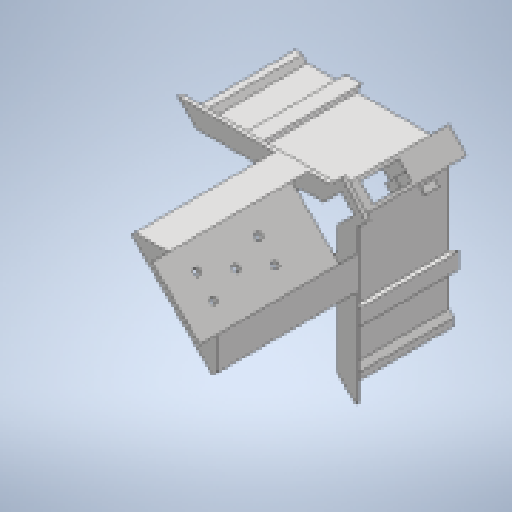
# Autodesk Inventor part: Kicker
Saved by Autodesk Inventor 2025.1 (Build 291241000, 241)
## iProperties
Created: 2025-05-21
Part Number: Kicker
Material: Generic
Document SubType Name: Modeling
Designer: User
Density: 1 g/cm^3
Appearance: Default
Author: User
Autodesk Inventor part; units mm, degrees
ref_plane "YZ Plane" through (0, 0, 0) normal (1, 0, 0) x (0, 1, 0)
sketch "Sketch1" plane through (0, 0, 0) normal (0, 0, 1) x (1, 0, 0)
  line L0 (-95.1092, -28.5) -> (-84.7092, -28.5) projected
  line L1 (-92.4092, -34) -> (-95.1092, -28.5) projected
  line L2 (-84.7092, -28.5) -> (-87.4092, -34) projected
  line L3 (-44.9455, -34) -> (-87.4092, -34) projected
  line L4 (-44.9455, -34) -> (-34.1024, -23.1569) projected
  line L5 (-34.1024, -23.1569) -> (-23.5803, -34.5602) projected
  line L6 (-34, -44.9799) -> (-23.5803, -34.5602) projected
  line L7 (-34, -87.4092) -> (-34, -44.9799) projected
  line L8 (-34, -87.4092) -> (-28.5, -84.7092) projected
  line L9 (-28.5, -84.7092) -> (-28.5, -95.1092) projected
  line L10 (-28.5, -95.1092) -> (-34, -92.4092) projected
  line L11 (-131.4592, -24.1043) -> (-125.0635, -30.5) projected
  line L12 (-121.2635, -34.3) -> (-91.9277, -34.3)
  line L13 (-91.9277, -34.3) -> (-94.6277, -28.8)
  line L14 (-94.6277, -28.8) -> (-85.1907, -28.8)
  line L15 (-85.1907, -28.8) -> (-87.8907, -34.3)
  line L16 (-87.8907, -34.3) -> (-44.8212, -34.3)
  line L17 (-44.8212, -34.3) -> (-34.111, -23.5898)
  line L18 (-34.111, -23.5898) -> (-23.9962, -34.5518)
  line L19 (-23.9962, -34.5518) -> (-34.3, -44.8556)
  line L20 (-34.3, -44.8556) -> (-34.3, -87.8907)
  line L21 (-34.3, -87.8907) -> (-28.8, -85.1907)
  line L22 (-28.8, -85.1907) -> (-28.8, -94.6277)
  line L23 (-28.8, -94.6277) -> (-34.3, -91.9277)
  line L24 (-34.3, -91.9277) -> (-34.3, -121.2635)
  line L25 (-36.8, -118.7635) -> (-36.8, -87.9155)
  line L26 (-36.8, -91.9029) -> (-36.8, -44.5272)
  line L27 (-44.4928, -36.8) -> (-91.9029, -36.8)
  line L28 (-87.9155, -36.8) -> (-118.7635, -36.8)
  line L29 (-34.3, -121.2635) -> (-36.8, -118.7635)
  line L30 (-121.2635, -34.3) -> (-118.7635, -36.8)
  line L31 (-43.9928, -36.3) -> (-34.169, -26.4762)
  line L32 (-34.169, -26.4762) -> (-26.769, -34.4961)
  line L33 (-26.769, -34.4961) -> (-36.3, -44.0272)
  line L34 (-43.9928, -36.3) -> (-44.4928, -36.8)
  line L35 (-36.3, -44.0272) -> (-36.8, -44.5272)
  point P0 (0, 0)
  dimension "d1" = 2.5
  constraints: 48 end point, 3 point on line, 1 parallel, 10 other
  measures "d1" distance between parallel lines of L12 L28
ref_plane "Work Plane1" through (-125.0635, -34, -60.4376) normal (0, 0, -1) x (0, 1, 0)
extrude "Extrusion1" add sketch "Sketch1" against normal up to surface (60.4376 mm away)
sketch "Sketch2" plane through (0, 0, 0) normal (0, 0, 1) x (1, 0, 0)
  line L0 (-91.9277, -34.3) -> (-121.2635, -34.3) projected
  line L1 (-94.6277, -28.8) -> (-91.9277, -34.3) projected
  line L2 (-85.1907, -28.8) -> (-94.6277, -28.8) projected
  line L3 (-87.8907, -34.3) -> (-85.1907, -28.8) projected
  line L4 (-44.8212, -34.3) -> (-87.8907, -34.3) projected
  line L5 (-34.111, -23.5898) -> (-44.8212, -34.3) projected
  line L6 (-23.9962, -34.5518) -> (-34.111, -23.5898) projected
  line L7 (-34.3, -44.8556) -> (-23.9962, -34.5518) projected
  line L8 (-34.3, -87.8907) -> (-34.3, -44.8556) projected
  line L9 (-28.8, -85.1907) -> (-34.3, -87.8907) projected
  line L10 (-28.8, -94.6277) -> (-28.8, -85.1907) projected
  line L11 (-34.3, -91.9277) -> (-28.8, -94.6277) projected
  line L12 (-34.3, -121.2635) -> (-34.3, -91.9277) projected
  line L13 (-31.3, -121.2635) -> (-31.3, -96.7425)
  line L14 (-31.3, -96.7425) -> (-25.8, -99.4425)
  line L15 (-25.8, -99.4425) -> (-25.8, -80.376)
  line L16 (-25.8, -80.376) -> (-31.3, -83.076)
  line L17 (-31.3, -83.076) -> (-31.3, -46.0983)
  line L18 (-31.3, -46.0983) -> (-19.8371, -34.6354)
  line L19 (-19.8371, -34.6354) -> (-34.0241, -19.2602)
  line L20 (-34.0241, -19.2602) -> (-46.0639, -31.3)
  line L21 (-46.0639, -31.3) -> (-83.076, -31.3)
  line L22 (-83.076, -31.3) -> (-80.376, -25.8)
  line L23 (-80.376, -25.8) -> (-99.4425, -25.8)
  line L24 (-99.4425, -25.8) -> (-96.7425, -31.3)
  line L25 (-96.7425, -31.3) -> (-121.2635, -31.3)
  line L26 (-131.4592, -24.1043) -> (-125.0635, -30.5) projected
  line L27 (-121.2635, -31.3) -> (-124.2635, -31.3)
  line L28 (-124.2635, -31.3) -> (-118.7635, -36.8)
  line L29 (-118.7635, -36.8) -> (-44.4928, -36.8) projected
  line L30 (-118.7635, -36.8) -> (-44.4928, -36.8)
  line L31 (-34.169, -26.4762) -> (-26.769, -34.4961) projected
  line L32 (-44.4928, -36.8) -> (-34.169, -26.4762)
  line L33 (-34.169, -26.4762) -> (-26.769, -34.4961)
  line L34 (-26.769, -34.4961) -> (-36.7828, -44.51)
  line L35 (-36.7828, -44.51) -> (-36.7828, -118.7807)
  line L36 (-36.7828, -118.7807) -> (-31.3, -124.2635)
  line L37 (-31.3, -124.2635) -> (-31.3, -121.2635)
  point P0 (0, 0)
  point P1 (-121.5635, -34)
  dimension "d5" = 3
  constraints: 45 end point, 3 point on line, 2 horizontal, 2 parallel, 2 perpendicular, 1 collinear, 12 other
  measures "d5" distance between parallel lines of L12 L13
extrude "Extrusion2" add sketch "Sketch2" along normal blind 2.5
sketch "Sketch3" plane through (0, 0, 0) normal (0, 0, -1) x (-1, 0, 0)
  line L0 (124.2635, -31.3) -> (121.2635, -34.3) projected
  line L1 (96.7425, -31.3) -> (124.2635, -31.3) projected
  line L2 (91.9277, -34.3) -> (121.2635, -34.3) projected
  line L3 (116.6137, -34) -> (120.1137, -30.5) projected
  line L4 (117.0209, -34.3) -> (120.0209, -31.3)
  line L5 (30.5, -120.1137) -> (34, -116.6137) projected
  line L6 (31.3, -120.0209) -> (34.3, -117.0209)
  line L7 (34.3, -121.2635) -> (34.3, -91.9277) projected
  line L8 (34.3, -121.2635) -> (31.3, -124.2635) projected
  line L9 (31.3, -124.2635) -> (31.3, -96.7425) projected
  point P0 (0, 0)
  dimension "d8" = 0.5
  dimension "d9" = 0.5
  constraints: 4 end point, 4 point on line, 2 parallel
  measures "d8" distance between parallel lines of L3 L4
  measures "d9" distance between parallel lines of L5 L6
extrude "Extrusion3" add sketch "Sketch3" along normal up to surface (60.4376 mm away)
fillet "Fillet1" radius 4 4 edges at (-118.7635, -36.8, -30.2188) (-118.7635, -36.8, 1.25) (-36.8, -118.7635, -30.2188) (-36.7828, -118.7807, 1.25)
sketch "Sketch4" plane through (0, 0, 2.5) normal (0, 0, 1) x (1, 0, 0)
  line L0 (-46.0639, -31.3) -> (-83.076, -31.3) projected
  line L1 (-96.7425, -31.3) -> (-124.2635, -31.3) projected
  line L2 (-80.376, -25.8) -> (-99.4425, -25.8) projected
  line L3 (-83.076, -31.3) -> (-80.376, -25.8) projected
  line L4 (-99.4425, -25.8) -> (-96.7425, -31.3) projected
  line L5 (-34.0241, -19.2602) -> (-46.0639, -31.3) projected
  line L6 (-124.2635, -31.3) -> (-119.9351, -35.6284) projected
  line L7 (-131.4592, -24.1043) -> (-125.0635, -30.5) projected
  line L8 (-99.4425, -25.8) -> (-129.7635, -25.8)
  line L9 (-129.7635, -25.8) -> (-124.2635, -31.3)
  line L10 (-124.2635, -31.3) -> (-96.7425, -31.3)
  line L11 (-91.9277, -34.3) -> (-117.0209, -34.3) projected
  line L12 (-96.7425, -31.3) -> (-99.4425, -25.8)
  line L13 (-83.076, -31.3) -> (-80.376, -25.8)
  line L14 (-80.376, -25.8) -> (-99.4425, -25.8) projected
  line L15 (-80.376, -25.8) -> (-40.5639, -25.8)
  line L16 (-40.5639, -25.8) -> (-46.0639, -31.3)
  line L17 (-46.0639, -31.3) -> (-83.076, -31.3) projected
  line L18 (-46.0639, -31.3) -> (-83.076, -31.3)
  line L19 (-83.076, -31.3) -> (-80.376, -25.8) projected
  line L20 (-83.076, -31.3) -> (-80.376, -25.8)
  line L21 (-25.8, -80.376) -> (-31.3, -83.076) projected
  line L22 (-31.3, -83.076) -> (-31.3, -46.0983) projected
  line L23 (-31.3, -46.0983) -> (-19.8371, -34.6354) projected
  line L24 (-31.3, -96.7425) -> (-25.8, -99.4425) projected
  line L25 (-31.3, -124.2635) -> (-31.3, -96.7425) projected
  line L26 (-35.6112, -119.9523) -> (-31.3, -124.2635) projected
  line L27 (-30.5, -125.0635) -> (-24.1043, -131.4592) projected
  line L28 (-25.8, -99.4425) -> (-25.8, -129.7635)
  line L29 (-25.8, -129.7635) -> (-31.3, -124.2635)
  line L30 (-31.3, -124.2635) -> (-31.3, -96.7425)
  line L31 (-31.3, -96.7425) -> (-25.8, -99.4425)
  line L32 (-25.8, -80.376) -> (-31.3, -83.076)
  line L33 (-31.3, -83.076) -> (-31.3, -46.0983)
  line L34 (-25.8, -80.376) -> (-25.8, -40.5983)
  line L35 (-25.8, -40.5983) -> (-31.3, -46.0983)
  line L36 (-34.3, -44.8556) -> (-23.9962, -34.5518) projected
  line L37 (-31.3, -46.0983) -> (-31.3, -83.076)
  line L38 (-34.3, -87.8907) -> (-34.3, -44.8556) projected
  line L39 (-25.8, -80.376) -> (-31.3, -83.076)
  point P0 (0, 0)
  constraints: 38 end point, 7 collinear, 5 parallel, 5 point on line, 2 vertical, 1 horizontal
extrude "Extrusion4" add sketch "Sketch4" against normal up to surface (2.5 mm away)
sketch "Sketch5" plane through (0, 0, 2.5) normal (0, 0, 1) x (1, 0, 0)
  line L0 (-56.2709, -42.724) -> (-60.815, -38.18) projected
  line L1 (-56.235, -42.7599) -> (-42.5671, -56.4279) projected
  line L2 (-37.9871, -61.0078) -> (-42.5312, -56.4638) projected
  line L3 (-37.9871, -61.0078) -> (-60.815, -38.18)
  line L4 (-60.815, -38.18) -> (-62.9363, -40.3013)
  line L5 (-62.9363, -40.3013) -> (-40.1085, -63.1291)
  line L6 (-40.1085, -63.1291) -> (-37.9871, -61.0078)
  point P0 (0, 0)
  dimension "d15" = 3
  constraints: 8 end point, 2 parallel, 1 collinear, 1 perpendicular
  measures "d15" distance of L4.end L0.end
ref_plane "Work Plane2" through (-59.6026, -59.7955, 84.008) normal (0, 0, 1) x (0.7071068, -0.7071068, 0)
extrude "Extrusion5" add sketch "Sketch5" along normal up to surface (81.508 mm away)
sketch "Sketch6" plane through (-62.9363, -40.3013, 84.008) normal (-0.7071068, -0.7071068, 0) x (-0.7071068, 0.7071068, 0)
  spline S0 degree 3 poles (-18.1417, 35.1354) (-18.1417, 35.3868) (-18.0914, 35.6547) (-17.8872, 36.1474) (-17.7334, 36.3722) (-17.3785, 36.7271) (-17.1537, 36.8809) (-16.661, 37.0851) (-16.3931, 37.1354) (-15.8903, 37.1354) (-15.6224, 37.0851) (-15.1297, 36.8809) (-14.9049, 36.7271) (-14.55, 36.3722) (-14.3962, 36.1474) (-14.192, 35.6547) (-14.1417, 35.3868) (-14.1417, 34.884) (-14.192, 34.6161) (-14.3962, 34.1234) (-14.55, 33.8986) (-14.9049, 33.5437) (-15.1297, 33.3899) (-15.6224, 33.1857) (-15.8903, 33.1354) (-16.3931, 33.1354) (-16.661, 33.1857) (-17.1537, 33.3899) (-17.3785, 33.5437) (-17.7334, 33.8986) (-17.8872, 34.1234) (-18.0914, 34.6161) (-18.1417, 34.884) (-18.1417, 35.1354) knots 0 0 0 0 0.07541 0.07541 0.150821 0.150821 0.226231 0.226231 0.30164 0.30164 0.37705 0.37705 0.45246 0.45246 0.52787 0.52787 0.603281 0.603281 0.678691 0.678691 0.754101 0.754101 0.829511 0.829511 0.904921 0.904921 0.980331 0.980331 1.055741 1.055741 1.131151 1.131151 1.206562 1.206562 1.206562 1.206562 projected
  circle A0 centre (-9.2456, 17.1903) radius 2 projected
  circle A1 centre (-23.0378, 17.1903) radius 2 projected
  circle A2 centre (-23.0378, 53.0805) radius 2 projected
  circle A3 centre (-9.2456, 53.0805) radius 2 projected
  point P0 (-16.0053, 84.008)
  point P1 (-18.1417, 35.1354)
extrude "Extrusion6" cut sketch "Sketch6" against normal blind 10
sketch "Sketch7" plane through (-37.9871, -61.0078, 84.008) normal (0, 0, 1) x (0.7071068, 0.7071068, 0)
  line L0 (-40, -57.2352) -> (23.0493, 5.8141) projected
  line L1 (23.0737, 26.7177) -> (-40, 89.7914) projected
  line L2 (0, 32.2834) -> (0, 0) projected
  line L3 (-3, 0) -> (-3, 32.2834) projected
  line L4 (0, 49.7914) -> (0, -17.2352)
  line L5 (0, -17.2352) -> (-3, -17.2352)
  line L6 (-3, -17.2352) -> (-3, 49.7914)
  line L7 (-3, 49.7914) -> (0, 49.7914)
  line L8 (-3, 32.2834) -> (0, 32.2834) projected
  line L9 (0, 32.2834) -> (-3, 32.2834)
  line L10 (-3, 32.2834) -> (-3, 0)
  line L11 (0, 0) -> (-3, 0) projected
  line L12 (0, 0) -> (-3, 0)
  point P0 (70, 16.2781)
  point P1 (0, 0)
  point P2 (-3, 0)
  point P3 (-3, 32.2834)
  point P4 (0, 32.2834)
  constraints: 14 end point, 3 equal length, 3 perpendicular, 2 point on line, 1 vertical
extrude "Extrusion7" add sketch "Sketch7" against normal up to surface (81.508 mm away) contours L8 L6 L7 L4 | L4 L5 L6 L11
sketch "Sketch8" plane through (-25.8, -73.1949, 84.008) normal (0, 0, 1) x (0.7071068, 0.7071068, 0)
  arc A0 (7.1422, 21.3881) -> (31.9738, 21.3881) centre (19.558, 33.3769) ccw projected
  arc A1 (29.0311, 47.8041) -> (10.0849, 47.8041) centre (19.558, 33.3769) ccw projected
  line L0 (0, 0) -> (0, 67.0266) projected
  line L1 (19.558, 16.1176) -> (0, 16.1176)
  line L2 (19.558, 50.6362) -> (0, 50.6362)
  line L3 (19.558, 13.6176) -> (0, 13.6176)
  line L4 (19.558, 53.1362) -> (0, 53.1362)
  line L5 (19.558, 56.1362) -> (0, 56.1362)
  line L6 (19.558, 10.6176) -> (0, 10.6176)
  line L7 (0, 0) -> (23.0493, 23.0493) projected
  line L8 (23.0737, 43.9529) -> (0, 67.0266) projected
  line L9 (0, 67.0266) -> (0, 53.1362)
  line L10 (0, 67.0266) -> (0, 51.4702) projected
  line L11 (0, 67.0266) -> (13.8904, 53.1362)
  line L12 (13.6176, 13.6176) -> (0, 0)
  point P0 (70, 33.5133)
  point P1 (0, 13.6176)
  point P2 (0, 53.1362)
  dimension "d22" = 2.5
  dimension "d23" = 2.5
  dimension "d24" = 3
  dimension "d25" = 3
  constraints: 18 end point, 6 point on line, 4 parallel, 2 collinear, 2 perpendicular, 2 point on circle
  measures "d22" distance between parallel lines of L1 L3
  measures "d23" distance between parallel lines of L2 L4
  measures "d24" distance between parallel lines of L4 L5
  measures "d25" distance between parallel lines of L3 L6
extrude "Extrusion8" add sketch "Sketch8" against normal up to surface (81.508 mm away) contours L7 L6 L0 L3 | L7 L0 L6 | L4 L0 L5 L8 | L5 L0 L8
sketch "Sketch9" plane through (0, 0, 0) normal (0, 0, 1) x (1, 0, 0)
  arc A0 (-36.8, -117.1066) -> (-35.6284, -119.9351) centre (-32.8, -117.1066) ccw projected
  line L0 (-35.6284, -119.9351) -> (-35.6112, -119.9523) projected
  arc A1 (-36.7828, -117.1238) -> (-35.6112, -119.9523) centre (-32.7828, -117.1238) ccw projected
  line L1 (-36.7828, -117.1238) -> (-36.7828, -44.51) projected
  line L2 (-36.7828, -44.51) -> (-36.8, -44.5272) projected
  line L3 (-36.8, -44.5272) -> (-36.8, -117.1066) projected
  arc A2 (-36.8, -117.1066) -> (-35.6284, -119.9351) centre (-32.8, -117.1066) ccw projected
  line L4 (-35.6284, -119.9351) -> (-35.6112, -119.9523) projected
  arc A3 (-36.7828, -117.1238) -> (-35.6112, -119.9523) centre (-32.7828, -117.1238) ccw projected
  line L5 (-36.7828, -117.1238) -> (-36.7828, -44.51) projected
  line L6 (-36.7828, -44.51) -> (-36.8, -44.5272) projected
  line L7 (-36.8, -44.5272) -> (-36.8, -117.1066) projected
  point P0 (0, 0)
extrude "Extrusion9" add sketch "Sketch9" along normal up to surface (2.5 mm away)
sketch "Sketch10" plane through (-25.8, -73.1949, 84.008) normal (0.7071068, -0.7071068, 0) x (-0.7071068, -0.7071068, 0)
  circle A0 centre (18.28, 77.1107) radius 2.6 projected
  arc A1 (11.2777, 84.4585) -> (25.2659, 84.4741) centre (18.28, 77.1107) ccw projected
  circle A2 centre (18.28, 77.1107) radius 2.4
  circle A3 centre (18.28, 77.1107) radius 2.5
  circle A4 centre (18.28, 77.1107) radius 5.5
  point P0 (-70, 84.008)
  dimension "d30" = 4.8
  dimension "d31" = 5
  dimension "d32" = 3
  constraints: 3 centre point, 2 coincident
  measures "d30" diameter of A2
  measures "d31" diameter of A3
  measures "d32" radial gap between concentric circles of A3 A4
extrude "Extrusion10" add sketch "Sketch10" against normal blind 10 contours A0 | A3 | A4
sketch "Sketch11" plane through (-45.797, -79.0498, 6.8973) normal (-0.7071068, 0.7071068, 0) x (-0.7071068, -0.7071068, 0)
  circle A0 centre (0, 0) radius 5.5 projected
  point P0 (-88.28, -6.8973)
extrude "Extrusion11" add sketch "Sketch11" along normal blind 8.25
sketch "Sketch12" plane through (-25.8, -73.1949, 84.008) normal (0.7071068, -0.7071068, 0) x (0, 0, -1)
  arc A0 (81.508, -14.9764) -> (81.889, -15.5563) centre (77.1107, -18.28) ccw projected
  circle A1 centre (77.1107, -18.28) radius 5.5 projected
  point P0 (84.008, 70)
  point P1 (81.889, -15.5563)
  point P2 (81.508, -14.9764)
extrude "Extrusion12" cut sketch "Sketch12" against normal blind 16.75
sketch "Sketch13" plane through (-51.6306, -73.2162, 6.8973) normal (-0.7071068, 0.7071068, 0) x (-0.7071068, -0.7071068, 0)
  circle A0 centre (0, 0) radius 5.5 projected
  point P0 (-88.28, -6.8973)
extrude "Extrusion13" add sketch "Sketch13" against normal blind 4
sketch "Sketch14" plane through (-48.8022, -76.0446, 6.8973) normal (0.7071068, -0.7071068, 0) x (-0.7071068, -0.7071068, 0)
  circle A0 centre (0, 0) radius 5.5 projected
  circle A1 centre (0, 0) radius 6.5
  point P0 (-88.28, 6.8973)
  dimension "d41" = 13
  constraints: 1 centre point, 1 coincident
  measures "d41" diameter of A1
extrude "Extrusion14" add sketch "Sketch14" against normal blind 4
sketch "Sketch15" plane through (-48.8022, -76.0446, 6.8973) normal (0.7071068, -0.7071068, 0) x (-0.7071068, -0.7071068, 0)
  circle A0 centre (0, 0) radius 6.5 projected
  circle A1 centre (0, 0) radius 4.5
  point P0 (-88.28, 6.8973)
  dimension "d44" = 9
  constraints: 1 centre point, 1 coincident
  measures "d44" diameter of A1
extrude "Extrusion15" add sketch "Sketch15" along normal blind 4
sketch "Sketch16" plane through (-48.8022, -76.0446, 6.8973) normal (0.7071068, -0.7071068, 0) x (-0.7071068, -0.7071068, 0)
  circle A0 centre (0, 0) radius 4.5 projected
  circle A1 centre (0, 0) radius 2.35
  point P0 (-88.28, 6.8973)
  dimension "d47" = 4.7
  constraints: 1 centre point, 1 coincident
  measures "d47" diameter of A1
extrude "Extrusion16" cut sketch "Sketch16" against normal blind 4 contours A1
ref_plane "Work Plane3" through (-73.1974, -51.6494, 6.8973) normal (-0.7071068, 0.7071068, 0) x (-0.7071068, -0.7071068, 0)
sketch "Sketch17" plane through (-73.1974, -51.6494, 6.8973) normal (-0.7071068, 0.7071068, 0) x (-0.7071068, -0.7071068, 0)
  circle A0 centre (0, 0) radius 6.5 projected
  circle A1 centre (0, 0) radius 2.35
  point P0 (-88.28, -6.8973)
  dimension "d51" = 4.7
  constraints: 1 centre point, 1 coincident
  measures "d51" diameter of A1
extrude "Extrusion17" add sketch "Sketch17" along normal blind 8
sketch "Sketch19" plane through (-45.9738, -78.873, 6.8973) normal (0.7071068, -0.7071068, 0) x (-0.7071068, -0.7071068, 0)
  circle A0 centre (0, 0) radius 6.5 projected
  line L0 (-15.28, -77.1107) -> (-15.28, 4.3973) projected
  line L1 (0, -6.5) -> (-15.28, -6.5)
  line L2 (0, 6.5) -> (-15.28, 6.5)
  line L3 (-15.28, -6.5) -> (-15.28, 6.5)
  point P0 (-88.28, 6.8973)
  point P1 (-15.28, 4.3973)
  constraints: 6 end point, 2 perpendicular, 2 point on circle, 1 horizontal, 1 point on line, 1 tangent
extrude "Extrusion18" add sketch "Sketch19" against normal blind 8 contours A0 L1 L0 L3 L2
sketch "Sketch20" plane through (-36.8, -66.4376, 0.3973) normal (0.7071068, 0.7071068, 0) x (-0.7071068, 0.7071068, 0)
  line L0 (0, 2.1027) -> (5.6937, 2.1027) projected
  line L1 (0, 0) -> (0, 2.1027) projected
  line L2 (0, 0) -> (5.6937, 0) projected
  line L3 (5.6937, 2.1027) -> (5.6937, 0) projected
  point P0 (20.9569, -0.3973)
extrude "Extrusion19" add sketch "Sketch20" against normal up to surface surface through (-36.8, -118.7635, 0) normal (-1, 0, 0)
sketch "Sketch21" plane through (-78.8542, -45.9926, 6.8973) normal (-0.7071068, 0.7071068, 0) x (-0.7071068, -0.7071068, 0)
  circle A0 centre (0, 0) radius 6.5 projected
  line L0 (-15.28, 77.1107) -> (-15.28, -4.3973) projected
  line L1 (0, 6.5) -> (-15.28, 6.5)
  circle A1 centre (0, 0) radius 6.5 projected
  line L2 (0, -6.5) -> (-15.28, -6.5)
  line L3 (-15.28, -6.5) -> (-15.28, 6.5)
  point P0 (-88.28, -6.8973)
  constraints: 6 end point, 2 horizontal, 2 perpendicular, 1 point on circle, 1 point on line, 2 other
extrude "Extrusion20" add sketch "Sketch21" against normal blind 8 contours A0 L2 L3 L0 L1
sketch "Sketch22" plane through (-62.3928, -40.8448, 0.3973) normal (0.7071068, 0.7071068, 0) x (-0.7071068, 0.7071068, 0)
  line L0 (0, 2.1027) -> (5.7202, 2.1027) projected
  line L1 (0, 0) -> (0, 2.1027) projected
  line L2 (5.7202, 0) -> (0, 0) projected
  line L3 (5.7202, 2.1027) -> (5.7202, 0) projected
  point P0 (-15.2367, -0.3973)
extrude "Extrusion21" add sketch "Sketch22" along normal up to surface surface through (-44.4928, -36.8, 0) normal (0, -1, 0)
chamfer "Chamfer1" distance 15.25 angle 45 1 edges at (-65.2212, -38.0164, 13.3973)
chamfer "Chamfer2" distance 15.25 angle 45 1 edges at (-37.9976, -65.24, 13.3973)
chamfer "Chamfer3" distance 5 angle 45 4 edges at (-35.1692, -68.0684, 21.0223) (-35.1692, -68.0684, 7.9486) (-68.0496, -35.188, 7.9486) (-68.0496, -35.188, 21.0223)
sketch "Sketch24" plane through (-27.9213, -75.3163, 84.008) normal (-0.7071068, -0.7071068, 0) x (-0.7071068, 0.7071068, 0)
  line L0 (38.9529, 144.4456) -> (28.0493, 144.4456) projected
  line L1 (28.0493, 144.4456) -> (28.0493, 81.508) projected
  line L2 (38.9529, 81.508) -> (28.0493, 81.508) projected
  line L3 (38.9529, 144.4456) -> (38.9529, 81.508) projected
  line L4 (29.0493, 95.7123) -> (29.0493, 95.3686) projected
  line L5 (29.0493, 91.1447) -> (37.9533, 91.1447)
  line L6 (28.0493, 144.4456) -> (28.0493, 81.508) projected
  line L7 (38.9529, 91.1447) -> (28.0493, 91.1447)
  line L8 (28.0493, 91.1447) -> (28.0493, 113.6498)
  line L9 (28.0493, 113.6498) -> (38.9529, 113.6498)
  line L10 (38.9529, 113.6498) -> (38.9529, 91.1447)
  point P0 (33.5133, 84.008)
  point P1 (28.0493, 113.6498)
  point P2 (28.0493, 91.1447)
  point P3 (29.0493, 91.1447)
  point P4 (37.9533, 91.1447)
  dimension "d76" = 10.9036
  constraints: 10 end point, 2 horizontal, 2 parallel, 2 point on line, 1 perpendicular, 2 other
  measures "d76" distance of L8.end L9.end
extrude "Extrusion22" cut sketch "Sketch24" against normal through all contours L3 L7 L5 L1 L9
chamfer "Chamfer4" distance 2 angle 45 1 edges at (-30.469, -30.4862, -29.6418)
sketch "Sketch25" plane through (-44.8212, -34.3, -60.4376) normal (0, 0, -1) x (-1, 0, 0)
  line L0 (72.2854, -2.5) -> (-0.3284, -2.5) projected
  line L1 (-8.0212, -10.2272) -> (-8.0212, -82.8066) projected
  line L2 (28.3762, -17.3494) -> (13.5267, -2.5) projected
  line L3 (6.8094, -38.9162) -> (-8.0212, -24.0856) projected
  line L4 (-8.0212, -37.304) -> (-8.0212, -24.0856) projected
  line L5 (-6.1165, -37.304) -> (-8.0212, -37.304) projected
  line L6 (1.1525, -44.573) -> (-6.1165, -37.304) projected
  line L7 (1.1525, -44.573) -> (6.8094, -38.9162) projected
  line L8 (6.8094, -38.9162) -> (-8.0212, -24.0856) projected
  line L9 (13.5267, -2.5) -> (26.7639, -2.5) projected
  line L10 (28.3762, -17.3494) -> (13.5267, -2.5) projected
  line L11 (28.3762, -17.3494) -> (34.033, -11.6926) projected
  line L12 (26.7639, -4.4235) -> (34.033, -11.6926) projected
  line L13 (26.7639, -4.4235) -> (26.7639, -2.5) projected
  line L14 (28.3762, -17.3494) -> (13.5267, -2.5)
  line L15 (14.1982, -45.8817) -> (35.3435, -24.7363)
  line L16 (13.5267, -2.5) -> (35.5533, -24.5266)
  line L17 (35.5533, -24.5266) -> (13.9865, -46.0933)
  line L18 (13.9865, -46.0933) -> (-8.0212, -24.0856)
  line L19 (35.5533, -24.5266) -> (33.7855, -22.7588)
  line L20 (32.0178, -24.5266) -> (13.9865, -42.5578)
  line L21 (35.5533, -24.5266) -> (33.7855, -26.2943)
  line L22 (32.0178, -24.5266) -> (9.9912, -2.5)
  line L23 (13.9865, -46.0933) -> (15.7543, -44.3256)
  line L24 (13.9865, -42.5578) -> (-8.0212, -20.55)
  line L25 (-6.2535, -18.7823) -> (13.9865, -39.0223)
  line L26 (13.9865, -39.0223) -> (28.4822, -24.5266)
  line L27 (28.4822, -24.5266) -> (8.2234, -4.2678)
  line L28 (28.4822, -24.5266) -> (6.4557, -2.5)
  line L29 (13.9865, -39.0223) -> (-8.0212, -17.0145)
  point P0 (-44.8212, 34.3)
  point P1 (8.2234, -4.2678)
  point P2 (-6.2535, -18.7823)
  dimension "d82" = 2.5
  dimension "d83" = 2.5
  dimension "d84" = 2.5
  dimension "d85" = 2.5
  constraints: 32 end point, 11 point on line, 4 perpendicular, 1 collinear, 5 other
  measures "d82" distance of L16.end L19.end
  measures "d83" distance of L16.end L21.end
  measures "d84" distance of L17.end L23.end
  measures "d85" distance between parallel lines of L20 L26
extrude "Extrusion23" add sketch "Sketch25" against normal blind 8.5 contours L22 L20 L24 L1 L29 L25 L26 L27 L28 L0
sketch "Sketch26" plane through (-58.8078, -76.8578, -51.9376) normal (-0.7071068, -0.7071068, 0) x (-0.7071068, 0.7071068, 0)
  line L0 (23, 0) -> (23, 8.5) projected
  line L1 (23, 8.5) -> (23, 0) projected
  line L2 (2.5, 8.5) -> (2.5, 0) projected
  line L3 (2.5, 8.5) -> (2.5, 0) projected
  line L4 (0, 8.5) -> (25.5, 8.5) projected
  line L5 (0, 6) -> (25.5, 6)
  line L6 (23, 0) -> (2.5, 0)
  line L7 (2.5, 0) -> (2.5, 6)
  line L8 (2.5, 6) -> (23, 6)
  line L9 (23, 6) -> (23, 0)
  point P0 (12.7633, -51.9376)
  point P1 (23, 0)
  point P2 (23, 6)
  point P3 (2.5, 6)
  dimension "d88" = 2.5
  constraints: 10 end point, 3 parallel, 2 point on line, 1 horizontal, 1 perpendicular
  measures "d88" distance between parallel lines of L4 L5
extrude "Extrusion24" cut sketch "Sketch26" against normal blind 8.5 contours L6 L2 L5 L0
sketch "Sketch27" plane through (-58.8078, -73.3223, -57.9376) normal (0.7071068, 0.7071068, 0) x (0, 0, -1)
  line L0 (0, 20.5) -> (0, 0) projected
  line L1 (2.5, 0) -> (0, 0) projected
  line L2 (2.5, 20.5) -> (2.5, 0) projected
  line L3 (2.5, 20.5) -> (0, 20.5) projected
  point P0 (-57.9376, 10.2633)
extrude "Extrusion25" add sketch "Sketch27" along normal up to surface surface through (-26.769, -34.4961, 0) normal (-0.7349363, -0.6781362, 0)
sketch "Sketch28" plane through (-34.3, -48.8145, -57.9376) normal (0, 0, 1) x (1, 0, 0)
  line L0 (0, 0) -> (0, 3.9589) projected
  line L1 (0, 0) -> (10.7883, 10.7883) projected
  line L2 (8.8884, 12.8473) -> (10.7883, 10.7883) projected
  line L3 (0, 3.9589) -> (8.8884, 12.8473) projected
  line L4 (-10.5212, 14.5145) -> (-14.4769, 14.5145) projected
  line L5 (-1.2264, 23.8093) -> (-10.5212, 14.5145) projected
  line L6 (-3.1247, 25.8666) -> (-1.2264, 23.8093) projected
  line L7 (-14.4769, 14.5145) -> (-3.1247, 25.8666) projected
  point P0 (34.3, 48.8145)
extrude "Extrusion26" cut sketch "Sketch28" against normal blind 10
sketch "Sketch30" plane through (-36.7828, -44.51, 2.5) normal (-0.7071068, 0.7071068, 0) x (0.7071068, 0.7071068, 0)
  line L0 (-4.8237, 54.4376) -> (-38.4473, 54.4376) projected
  line L1 (14.1617, 34.1418) -> (16.1633, 32.1418) projected
  circle A0 centre (-30.7973, -4.3973) radius 2.35 projected
  line L2 (14.1617, 60.4376) -> (14.1617, 34.1418) projected
  circle A1 centre (-30.7973, -4.3973) radius 59.2164
  circle A2 centre (-30.7973, -4.3973) radius 61.7164
  line L3 (14.1617, 34.1418) -> (14.1617, 37.8826)
  line L4 (-0.0243, 2.5) -> (-0.0243, 60.4376) projected
  line L5 (-0.0243, 46.1952) -> (-0.0243, 49.0997)
  line L6 (-12.1596, 54.4376) -> (-24.0868, 54.4376)
  point P0 (57.4827, 2.5)
  dimension "d96" = 2.5
  constraints: 6 end point, 6 point on circle, 5 point on line, 2 centre point, 1 coincident
  measures "d96" radial gap between concentric circles of A1 A2
extrude "Extrusion27" add sketch "Sketch30" along normal blind 5 contours A2 L4 A1 L0 | A2 L2 A1 L4
sketch "Sketch31" plane through (-40.3183, -40.9745, 2.5) normal (-0.7071068, 0.7071068, 0) x (0.7071068, 0.7071068, 0)
  arc A0 (14.1617, 37.8826) -> (-12.1596, 54.4376) centre (-30.7973, -4.3973) ccw projected
  line L0 (-4.8237, 54.4376) -> (-38.4473, 54.4376) projected
  line L1 (-0.0243, 49.0997) -> (-0.0243, 60.4376) projected
  line L2 (-12.1596, 54.4376) -> (-0.0243, 54.4376)
  line L3 (-0.0243, 49.0997) -> (-0.0243, 54.4376)
  arc A1 (14.1617, 34.1418) -> (-24.0868, 54.4376) centre (-30.7973, -4.3973) ccw projected
  line L4 (-0.0243, 46.1952) -> (-0.0243, 49.0997)
  point P0 (57.4827, 2.5)
  point P1 (-4.8237, 54.4376)
  constraints: 6 end point, 2 point on line, 1 collinear, 1 point on circle, 1 vertical
extrude "Extrusion28" add sketch "Sketch31" against normal up to surface (12.2993 mm away)
sketch "Sketch32" plane through (-60.5755, -75.09, -51.9376) normal (-0.7071068, 0.7071068, 0) x (0.7071068, 0.7071068, 0)
  arc A0 (-25.35, -55.1572) -> (-25.35, -55.1572) centre (-25.35, -20.1572) ccw
  circle A1 centre (-25.35, -20.1572) radius 35
  circle A2 centre (-25.35, -20.1572) radius 37.5
  line L0 (14.3606, 0) -> (0, 0) projected
  line L1 (0, 8.5) -> (0, 0) projected
  point P0 (95.93, -51.9376)
  point P1 (0, 7.4766)
  point P2 (6.2718, 0)
  dimension "d101" = 2.5
  constraints: 2 centre point, 1 coincident, 1 vertical alignment, 5 other
  measures "d101" radial gap between concentric circles of A1 A2
extrude "Extrusion29" cut sketch "Sketch32" along normal mid plane 38.25 contours L0 L1 A0 | A0 L1 A2 L0 picked at (0.384, 2.2265) picked at (0.7683, 5.5405)
sketch "Sketch33" plane through (-36.8, -51.3145, -51.9376) normal (-0.7071068, 0.7071068, 0) x (0.7071068, 0.7071068, 0)
  line L0 (-19.2631, 0) -> (-27.3519, 0) projected
  arc A0 (-27.3519, 0) -> (-32.1027, 6) centre (-58.9737, -20.1572) ccw projected
  line L1 (-19.2631, 2.5) -> (-26.0093, 2.5)
  arc A1 (-26.0093, 2.5) -> (-30.3113, 7.7438) centre (-58.9737, -20.1572) ccw
  line L2 (-26.0093, 2.5) -> (-29.0923, 2.5)
  arc A2 (18.9854, -16.555) -> (4.7993, -5.3379) centre (-25.9737, -58.8349) ccw projected
  circle A3 centre (-25.9737, -58.8349) radius 2.35 projected
  arc A4 (-26.2634, 2.8653) -> (-19.2631, 2.5) centre (-25.9737, -58.8349) ccw
  line L3 (-27.3519, 0) -> (-7.3872, 0)
  line L4 (-26.9501, -51.9376) -> (-26.9501, 8.5) projected
  point P0 (62.3063, -51.9376)
  point P1 (-26.9501, 8.5)
  dimension "d104" = 2.5
  constraints: 7 point on circle, 6 end point, 2 centre point, 2 horizontal, 1 coincident, 2 other
  measures "d104" distance between parallel lines of L0 L1
extrude "Extrusion30" add sketch "Sketch33" along normal up to surface (9.7993 mm away) contours L0 L4 L2 L1 A4 L3 | L0 A0 L2 L4
sketch "Sketch34" plane through (-76.839, -58.8266, -60.4376) normal (-0.7071068, 0.7071068, 0) x (-0.7071068, -0.7071068, 0)
  arc A0 (-6.2718, 8.5) -> (0, 1.0234) centre (25.35, 28.6572) ccw projected
  line L0 (-31.1503, 8.5) -> (0, 8.5) projected
  line L1 (0, 0) -> (0, 8.5) projected
  point P0 (-95.93, 60.4376)
extrude "Extrusion31" cut sketch "Sketch34" against normal blind 10
sketch "Sketch35" plane through (-40.3183, -40.9745, 2.5) normal (-0.7071068, 0.7071068, 0) x (0.7071068, 0.7071068, 0)
  arc A0 (14.1617, 34.1418) -> (-24.0868, 54.4376) centre (-30.7973, -4.3973) ccw projected
  line L0 (14.1617, 34.1418) -> (14.1617, 37.8826) projected
  arc A1 (14.1617, 37.8826) -> (-0.0243, 49.0997) centre (-30.7973, -4.3973) ccw projected
  line L1 (-0.0243, 49.0997) -> (-0.0243, 54.4376) projected
  line L2 (-0.0243, 54.4376) -> (-12.2109, 54.4376) projected
  arc A2 (-12.2109, 54.4376) -> (-24.0868, 56.9376) centre (-30.7973, -4.3973) ccw projected
  line L3 (-33.9159, 56.9376) -> (-24.0868, 56.9376) projected
  arc A3 (-32.1756, 54.4376) -> (-33.9159, 56.9376) centre (-63.7973, 34.2804) ccw projected
  line L4 (-24.0868, 54.4376) -> (-32.1756, 54.4376) projected
  point P0 (57.4827, 2.5)
extrude "Extrusion32" add sketch "Sketch35" along normal up to surface (13.2007 mm away)
sketch "Sketch36" plane through (-52.3124, -34.3, -51.9376) normal (-0.7071068, 0.7071068, 0) x (-0.7071068, -0.7071068, 0)
  line L0 (-17.9233, 16.555) -> (-17.9233, 20.2958) projected
  line L1 (-17.9233, 20.2958) -> (-19.9249, 22.2958) projected
  line L2 (-19.9249, 22.2958) -> (-19.9249, 17.5046)
  arc A0 (-19.9249, 18.7009) -> (-17.9233, 16.555) centre (-4.2777, 31.2897) ccw
  point P0 (-61.2442, 51.9376)
  constraints: 2 end point, 2 point on circle, 1 centre point, 1 point on line, 1 vertical
extrude "Extrusion33" add sketch "Sketch36" against normal up to surface (18.2007 mm away)
sketch "Sketch37" plane through (-44.8212, -34.3, -60.4376) normal (0, 0, -1) x (-1, 0, 0)
  line L0 (-10.7102, 10.7102) -> (0, 0) projected
  line L1 (0, 0) -> (43.0694, 0) projected
  line L2 (-10.5212, -10.5556) -> (-20.825, -0.2518) projected
  line L3 (-10.5212, -53.5907) -> (-10.5212, -10.5556) projected
  line L4 (-15.8935, -5.1833) -> (-15.8935, -18.7166)
  line L5 (-15.8935, -18.7166) -> (-10.5212, -22.355)
  line L6 (-10.7102, 10.7102) -> (-7.1978, 23.2525)
  line L7 (-7.1978, 23.2525) -> (3.6115, 21.8141)
  line L8 (3.6115, 21.8141) -> (21.3317, 8.5)
  line L9 (21.3317, 8.5) -> (13.6408, 0)
  point P0 (-44.8212, 34.3)
  constraints: 12 end point, 3 point on line, 1 vertical
extrude "Extrusion34" cut sketch "Sketch37" against normal blind 44.75
sketch "Sketch38" plane through (-44.8212, -34.3, -60.4376) normal (0, 0, -1) x (-1, 0, 0)
  line L0 (12.5501, -37.5858) -> (5.5998, -30.6356) projected
  line L1 (-2.7977, -22.238) -> (5.5998, -30.6356) projected
  line L2 (-8.0212, -17.0145) -> (-2.7977, -22.238) projected
  line L3 (20.0955, -16.1399) -> (27.0458, -23.0901) projected
  line L4 (20.0955, -16.1399) -> (11.698, -7.7424) projected
  line L5 (11.698, -7.7424) -> (6.4557, -2.5) projected
  line L6 (13.9865, -42.5578) -> (32.0178, -24.5266) projected
  line L7 (-20.825, -0.2518) -> (-10.7102, 10.7102) projected
  line L8 (-8.0212, -10.2272) -> (-8.0212, -17.0145) projected
  line L9 (6.4557, -2.5) -> (-0.3284, -2.5) projected
  line L10 (-18.0523, -0.1961) -> (-8.0212, -10.2272) projected
  line L11 (-0.3284, -2.5) -> (-10.6522, 7.8238) projected
  line L12 (-10.6522, 7.8238) -> (-18.0523, -0.1961) projected
  line L13 (12.5501, -37.5858) -> (15.7543, -40.79)
  line L14 (12.5501, -37.5858) -> (27.0458, -23.0901) projected
  line L15 (27.0458, -23.0901) -> (30.25, -26.2943)
  point P0 (-44.8212, 34.3)
  constraints: 4 end point, 2 point on line, 1 perpendicular
extrude "Extrusion35" cut sketch "Sketch38" against normal blind 2.5
sketch "Sketch39" plane through (-44.8212, -34.3, -60.4376) normal (-0.7071068, 0.7071068, 0) x (0, 0, 1)
  arc A0 (25.055, 12.6262) -> (13.8379, -1.5598) centre (67.3349, -32.3329) ccw projected
  line L0 (13.8379, -1.5598) -> (8.5, -1.5598) projected
  line L1 (8.5, -6.3592) -> (8.5, -1.5598) projected
  line L2 (8.5, -6.3592) -> (8.5, -13.7464) projected
  ellipse E0 centre (39.7897, -1.0193) end of major axis (39.7897, 19.0633) minor radius 20.0826 (25.4733, 13.0645) -> (25.055, 12.6262) ccw projected
  line L3 (0, 12.6262) -> (25.055, 12.6262) projected
  line L4 (0, 13.0645) -> (25.4733, 13.0645) projected
  line L5 (0, 15.1465) -> (0, 0) projected
  line L6 (60.4376, 0) -> (0, 0) projected
  point P0 (60.4376, 55.9472)
  constraints: 1 other
body "Solid1"
